Autodesk Fusion 360 part; units mm, degrees
(part 4 of 12)
  spline S130 degree 5 poles (-15.9343, -68.6757) (-15.9205, -68.6585) (-15.8929, -68.6243) (-15.8515, -68.5729) (-15.7966, -68.5042) (-15.7284, -68.4182) (-15.6605, -68.332) (-15.593, -68.2456) (-15.5259, -68.1591) (-15.4592, -68.0723) (-15.3928, -67.9855) (-15.3269, -67.8984) (-15.2613, -67.8111) (-15.1961, -67.7237) (-15.1313, -67.6361) (-15.0669, -67.5484) (-15.0029, -67.4604) (-14.9393, -67.3723) (-14.8761, -67.284) (-14.8134, -67.1956) (-14.751, -67.1069) (-14.6891, -67.0181) (-14.6276, -66.9291) (-14.5665, -66.8399) (-14.5059, -66.7506) (-14.4456, -66.6611) (-14.3859, -66.5714) (-14.3265, -66.4815) (-14.2676, -66.3914) (-14.2092, -66.3012) (-14.1512, -66.2108) (-14.0937, -66.1202) (-14.0367, -66.0294) (-13.9801, -65.9385) (-13.924, -65.8473) (-13.8684, -65.756) (-13.8133, -65.6645) (-13.7587, -65.5728) (-13.7046, -65.481) (-13.651, -65.3889) (-13.5979, -65.2967) (-13.5453, -65.2043) (-13.4933, -65.1117) (-13.4418, -65.0189) (-13.3909, -64.9259) (-13.3405, -64.8327) (-13.2907, -64.7393) (-13.2415, -64.6458) (-13.1928, -64.552) (-13.1448, -64.4581) (-13.0974, -64.3639) (-13.0506, -64.2695) (-13.0044, -64.175) (-12.9589, -64.0802) (-12.9141, -63.9852) (-12.873, -63.8968) (-12.8413, -63.8272) (-12.8185, -63.7766) (-12.8044, -63.745) (-12.7989, -63.7326) knots -1 -1 -1 -1 -1 -1 -0.985714 -0.971429 -0.957143 -0.942857 -0.928571 -0.914286 -0.9 -0.885714 -0.871429 -0.857143 -0.842857 -0.828571 -0.814286 -0.8 -0.785714 -0.771429 -0.757143 -0.742857 -0.728571 -0.714286 -0.7 -0.685714 -0.671429 -0.657143 -0.642857 -0.628571 -0.614286 -0.6 -0.585714 -0.571429 -0.557143 -0.542857 -0.528571 -0.514286 -0.5 -0.485714 -0.471429 -0.457143 -0.442857 -0.428571 -0.414286 -0.4 -0.385714 -0.371429 -0.357143 -0.342857 -0.328571 -0.314286 -0.3 -0.285714 -0.271429 -0.257143 -0.242857 -0.228571 -0.21931 -0.21931 -0.21931 -0.21931 -0.21931 -0.21931
  spline S131 degree 3 poles (-11.166, -62.8653) (-11.3583, -62.8311) (-11.5555, -62.8348) (-11.9372, -62.9176) (-12.1182, -62.9959) (-12.3924, -63.1847) (-12.4944, -63.278) (-12.6701, -63.4896) (-12.743, -63.607) (-12.7989, -63.7326) knots 0 0 0 0 0.058597 0.058597 0.117193 0.117193 0.158456 0.158456 0.199718 0.199718 0.199718 0.199718
  arc A66 (-11.166, -62.8653) -> (-11.0086, -62.893) centre (0, 0) ccw
  spline S132 degree 3 poles (-9.7708, -64.2666) (-9.7843, -64.0717) (-9.8358, -63.8814) (-10.0088, -63.5311) (-10.1287, -63.3746) (-10.3784, -63.1545) (-10.4935, -63.0781) (-10.7415, -62.959) (-10.8731, -62.9167) (-11.0086, -62.893) knots 0 0 0 0 0.058597 0.058597 0.117193 0.117193 0.158456 0.158456 0.199718 0.199718 0.199718 0.199718
  spline S133 degree 5 poles (-9.7708, -64.2666) (-9.7698, -64.2801) (-9.7674, -64.3146) (-9.7633, -64.3699) (-9.7573, -64.4461) (-9.749, -64.5433) (-9.7393, -64.6479) (-9.729, -64.7525) (-9.7179, -64.8572) (-9.7062, -64.9618) (-9.6939, -65.0665) (-9.6809, -65.1713) (-9.6673, -65.276) (-9.653, -65.3808) (-9.6381, -65.4855) (-9.6227, -65.5903) (-9.6066, -65.6951) (-9.5899, -65.7999) (-9.5727, -65.9048) (-9.555, -66.0096) (-9.5366, -66.1144) (-9.5177, -66.2192) (-9.4983, -66.3241) (-9.4783, -66.4289) (-9.4578, -66.5337) (-9.4368, -66.6386) (-9.4153, -66.7434) (-9.3932, -66.8482) (-9.3707, -66.953) (-9.3476, -67.0578) (-9.3241, -67.1626) (-9.3, -67.2674) (-9.2755, -67.3721) (-9.2505, -67.4769) (-9.225, -67.5816) (-9.199, -67.6863) (-9.1726, -67.791) (-9.1457, -67.8957) (-9.1183, -68.0004) (-9.0905, -68.105) (-9.0622, -68.2097) (-9.0335, -68.3143) (-9.0043, -68.4188) (-8.9747, -68.5234) (-8.9447, -68.6279) (-8.9142, -68.7324) (-8.8832, -68.8369) (-8.8519, -68.9413) (-8.8201, -69.0457) (-8.7879, -69.1501) (-8.7552, -69.2544) (-8.7222, -69.3587) (-8.6887, -69.463) (-8.6548, -69.5673) (-8.6205, -69.6715) (-8.5858, -69.7756) (-8.5577, -69.859) (-8.5365, -69.9214) (-8.5222, -69.9631) (-8.5151, -69.9839) knots 0.21931 0.21931 0.21931 0.21931 0.21931 0.21931 0.228571 0.242857 0.257143 0.271429 0.285714 0.3 0.314286 0.328571 0.342857 0.357143 0.371429 0.385714 0.4 0.414286 0.428571 0.442857 0.457143 0.471429 0.485714 0.5 0.514286 0.528571 0.542857 0.557143 0.571429 0.585714 0.6 0.614286 0.628571 0.642857 0.657143 0.671429 0.685714 0.7 0.714286 0.728571 0.742857 0.757143 0.771429 0.785714 0.8 0.814286 0.828571 0.842857 0.857143 0.871429 0.885714 0.9 0.914286 0.928571 0.942857 0.957143 0.971429 0.985714 1 1 1 1 1 1
  arc A67 (-8.5151, -69.9839) -> (-6.2215, -70.2249) centre (0, 0) ccw
  spline S134 degree 5 poles (-6.2215, -70.2249) (-6.2101, -70.2061) (-6.1875, -70.1683) (-6.1538, -70.1116) (-6.109, -70.036) (-6.0534, -69.9413) (-5.9981, -69.8465) (-5.9433, -69.7516) (-5.8889, -69.6565) (-5.8349, -69.5614) (-5.7813, -69.4661) (-5.7281, -69.3707) (-5.6753, -69.2752) (-5.6229, -69.1795) (-5.5709, -69.0838) (-5.5194, -68.9879) (-5.4682, -68.8919) (-5.4175, -68.7958) (-5.3672, -68.6996) (-5.3174, -68.6032) (-5.268, -68.5068) (-5.219, -68.4102) (-5.1705, -68.3135) (-5.1224, -68.2167) (-5.0748, -68.1198) (-5.0276, -68.0228) (-4.9809, -67.9256) (-4.9347, -67.8284) (-4.8889, -67.731) (-4.8436, -67.6335) (-4.7988, -67.5359) (-4.7544, -67.4382) (-4.7106, -67.3404) (-4.6672, -67.2424) (-4.6243, -67.1444) (-4.582, -67.0462) (-4.5401, -66.9479) (-4.4988, -66.8495) (-4.458, -66.751) (-4.4177, -66.6524) (-4.378, -66.5537) (-4.3388, -66.4549) (-4.3002, -66.3559) (-4.2621, -66.2569) (-4.2246, -66.1577) (-4.1877, -66.0584) (-4.1514, -65.959) (-4.1156, -65.8595) (-4.0805, -65.7599) (-4.0461, -65.6602) (-4.0122, -65.5603) (-3.979, -65.4604) (-3.9464, -65.3603) (-3.9145, -65.2601) (-3.8833, -65.1598) (-3.855, -65.0665) (-3.8333, -64.9932) (-3.8178, -64.9399) (-3.8082, -64.9067) (-3.8045, -64.8937) knots -1 -1 -1 -1 -1 -1 -0.985714 -0.971429 -0.957143 -0.942857 -0.928571 -0.914286 -0.9 -0.885714 -0.871429 -0.857143 -0.842857 -0.828571 -0.814286 -0.8 -0.785714 -0.771429 -0.757143 -0.742857 -0.728571 -0.714286 -0.7 -0.685714 -0.671429 -0.657143 -0.642857 -0.628571 -0.614286 -0.6 -0.585714 -0.571429 -0.557143 -0.542857 -0.528571 -0.514286 -0.5 -0.485714 -0.471429 -0.457143 -0.442857 -0.428571 -0.414286 -0.4 -0.385714 -0.371429 -0.357143 -0.342857 -0.328571 -0.314286 -0.3 -0.285714 -0.271429 -0.257143 -0.242857 -0.228571 -0.21931 -0.21931 -0.21931 -0.21931 -0.21931 -0.21931
  spline S135 degree 3 poles (-2.3082, -63.8075) (-2.5034, -63.8004) (-2.6981, -63.8315) (-3.0646, -63.9667) (-3.2329, -64.0694) (-3.4781, -64.2945) (-3.5662, -64.401) (-3.7108, -64.635) (-3.7667, -64.7614) (-3.8045, -64.8937) knots 0 0 0 0 0.058597 0.058597 0.117193 0.117193 0.158456 0.158456 0.199718 0.199718 0.199718 0.199718
  arc A68 (-2.3082, -63.8075) -> (-2.1484, -63.813) centre (0, 0) ccw
  spline S136 degree 3 poles (-0.7315, -65.001) (-0.772, -64.8099) (-0.8495, -64.6286) (-1.0696, -64.3058) (-1.2101, -64.1675) (-1.488, -63.9842) (-1.6126, -63.9247) (-1.8748, -63.8412) (-2.0109, -63.8177) (-2.1484, -63.813) knots 0 0 0 0 0.058597 0.058597 0.117193 0.117193 0.158456 0.158456 0.199718 0.199718 0.199718 0.199718
  spline S137 degree 5 poles (-0.7315, -65.001) (-0.7287, -65.0143) (-0.7215, -65.048) (-0.7097, -65.1022) (-0.6932, -65.1769) (-0.6714, -65.272) (-0.6473, -65.3742) (-0.6225, -65.4764) (-0.597, -65.5785) (-0.5708, -65.6805) (-0.544, -65.7824) (-0.5166, -65.8843) (-0.4885, -65.9862) (-0.4598, -66.0879) (-0.4305, -66.1896) (-0.4006, -66.2912) (-0.3701, -66.3928) (-0.339, -66.4942) (-0.3074, -66.5956) (-0.2752, -66.697) (-0.2425, -66.7982) (-0.2092, -66.8994) (-0.1753, -67.0005) (-0.141, -67.1016) (-0.1061, -67.2025) (-0.0707, -67.3034) (-0.0348, -67.4042) (0.0017, -67.5049) (0.0386, -67.6056) (0.076, -67.7061) (0.1139, -67.8066) (0.1523, -67.907) (0.1912, -68.0074) (0.2305, -68.1076) (0.2703, -68.2078) (0.3106, -68.3079) (0.3514, -68.4079) (0.3926, -68.5078) (0.4343, -68.6076) (0.4764, -68.7074) (0.5189, -68.8071) (0.5619, -68.9066) (0.6054, -69.0061) (0.6492, -69.1055) (0.6936, -69.2049) (0.7383, -69.3041) (0.7835, -69.4032) (0.829, -69.5023) (0.8751, -69.6013) (0.9215, -69.7002) (0.9683, -69.7989) (1.0156, -69.8976) (1.0632, -69.9962) (1.1113, -70.0948) (1.1598, -70.1932) (1.2086, -70.2915) (1.248, -70.3701) (1.2778, -70.429) (1.2977, -70.4683) (1.3077, -70.4879) knots 0.21931 0.21931 0.21931 0.21931 0.21931 0.21931 0.228571 0.242857 0.257143 0.271429 0.285714 0.3 0.314286 0.328571 0.342857 0.357143 0.371429 0.385714 0.4 0.414286 0.428571 0.442857 0.457143 0.471429 0.485714 0.5 0.514286 0.528571 0.542857 0.557143 0.571429 0.585714 0.6 0.614286 0.628571 0.642857 0.657143 0.671429 0.685714 0.7 0.714286 0.728571 0.742857 0.757143 0.771429 0.785714 0.8 0.814286 0.828571 0.842857 0.857143 0.871429 0.885714 0.9 0.914286 0.928571 0.942857 0.957143 0.971429 0.985714 1 1 1 1 1 1
  arc A69 (1.3077, -70.4879) -> (3.6125, -70.4074) centre (0, 0) ccw
  spline S138 degree 5 poles (3.6125, -70.4074) (3.6211, -70.3871) (3.6382, -70.3466) (3.6638, -70.2857) (3.6976, -70.2046) (3.7395, -70.1031) (3.781, -70.0015) (3.8221, -69.8999) (3.8627, -69.7982) (3.903, -69.6965) (3.9428, -69.5946) (3.9822, -69.4928) (4.0212, -69.3908) (4.0598, -69.2888) (4.0979, -69.1868) (4.1356, -69.0847) (4.1729, -68.9825) (4.2097, -68.8803) (4.2461, -68.778) (4.2821, -68.6756) (4.3176, -68.5733) (4.3526, -68.4708) (4.3872, -68.3683) (4.4214, -68.2658) (4.455, -68.1632) (4.4882, -68.0605) (4.521, -67.9578) (4.5532, -67.855) (4.585, -67.7522) (4.6163, -67.6494) (4.6471, -67.5465) (4.6774, -67.4436) (4.7072, -67.3406) (4.7366, -67.2376) (4.7654, -67.1345) (4.7936, -67.0314) (4.8214, -66.9283) (4.8486, -66.8251) (4.8753, -66.7219) (4.9015, -66.6186) (4.9271, -66.5153) (4.9521, -66.412) (4.9766, -66.3086) (5.0005, -66.2052) (5.0239, -66.1018) (5.0466, -65.9983) (5.0688, -65.8949) (5.0903, -65.7913) (5.1112, -65.6878) (5.1314, -65.5843) (5.1511, -65.4807) (5.17, -65.3771) (5.1884, -65.2735) (5.206, -65.1698) (5.2229, -65.0662) (5.238, -64.9698) (5.2493, -64.8941) (5.2573, -64.8392) (5.2621, -64.805) (5.264, -64.7916) knots -1 -1 -1 -1 -1 -1 -0.985714 -0.971429 -0.957143 -0.942857 -0.928571 -0.914286 -0.9 -0.885714 -0.871429 -0.857143 -0.842857 -0.828571 -0.814286 -0.8 -0.785714 -0.771429 -0.757143 -0.742857 -0.728571 -0.714286 -0.7 -0.685714 -0.671429 -0.657143 -0.642857 -0.628571 -0.614286 -0.6 -0.585714 -0.571429 -0.557143 -0.542857 -0.528571 -0.514286 -0.5 -0.485714 -0.471429 -0.457143 -0.442857 -0.428571 -0.414286 -0.4 -0.385714 -0.371429 -0.357143 -0.342857 -0.328571 -0.314286 -0.3 -0.285714 -0.271429 -0.257143 -0.242857 -0.228571 -0.21931 -0.21931 -0.21931 -0.21931 -0.21931 -0.21931
  spline S139 degree 3 poles (6.5945, -63.5077) (6.4003, -63.5279) (6.2118, -63.5858) (5.8676, -63.7707) (5.7153, -63.8958) (5.5038, -64.1529) (5.4314, -64.2706) (5.3208, -64.5225) (5.2831, -64.6554) (5.264, -64.7916) knots 0 0 0 0 0.058597 0.058597 0.117193 0.117193 0.158456 0.158456 0.199718 0.199718 0.199718 0.199718
  arc A70 (6.5945, -63.5077) -> (6.7536, -63.491) centre (0, 0) ccw
  spline S140 degree 3 poles (8.322, -64.4702) (8.2553, -64.2866) (8.1533, -64.1178) (7.8905, -63.8288) (7.7321, -63.7114) (7.4314, -63.5686) (7.2996, -63.527) (7.0285, -63.4808) (6.8903, -63.4765) (6.7536, -63.491) knots 0 0 0 0 0.058597 0.058597 0.117193 0.117193 0.158456 0.158456 0.199718 0.199718 0.199718 0.199718
  spline S141 degree 5 poles (8.322, -64.4702) (8.3266, -64.483) (8.3385, -64.5154) (8.3576, -64.5674) (8.3844, -64.6391) (8.4192, -64.7302) (8.4573, -64.8281) (8.4961, -64.9258) (8.5356, -65.0233) (8.5757, -65.1207) (8.6164, -65.218) (8.6578, -65.3151) (8.6997, -65.412) (8.7423, -65.5087) (8.7855, -65.6054) (8.8292, -65.7018) (8.8736, -65.7981) (8.9185, -65.8943) (8.9639, -65.9903) (9.0099, -66.0862) (9.0564, -66.1819) (9.1035, -66.2775) (9.151, -66.3729) (9.1991, -66.4681) (9.2477, -66.5633) (9.2968, -66.6582) (9.3464, -66.7531) (9.3965, -66.8477) (9.4471, -66.9423) (9.4981, -67.0367) (9.5497, -67.1309) (9.6017, -67.225) (9.6541, -67.3189) (9.707, -67.4127) (9.7604, -67.5064) (9.8142, -67.5999) (9.8685, -67.6932) (9.9232, -67.7864) (9.9784, -67.8795) (10.034, -67.9724) (10.09, -68.0652) (10.1464, -68.1578) (10.2033, -68.2503) (10.2606, -68.3427) (10.3183, -68.4348) (10.3764, -68.5269) (10.4349, -68.6188) (10.4938, -68.7105) (10.5532, -68.8021) (10.6129, -68.8936) (10.673, -68.9849) (10.7336, -69.0761) (10.7945, -69.1671) (10.8558, -69.2579) (10.9175, -69.3487) (10.9795, -69.4392) (11.0295, -69.5116) (11.0672, -69.5658) (11.0923, -69.6019) (11.105, -69.6199) knots 0.21931 0.21931 0.21931 0.21931 0.21931 0.21931 0.228571 0.242857 0.257143 0.271429 0.285714 0.3 0.314286 0.328571 0.342857 0.357143 0.371429 0.385714 0.4 0.414286 0.428571 0.442857 0.457143 0.471429 0.485714 0.5 0.514286 0.528571 0.542857 0.557143 0.571429 0.585714 0.6 0.614286 0.628571 0.642857 0.657143 0.671429 0.685714 0.7 0.714286 0.728571 0.742857 0.757143 0.771429 0.785714 0.8 0.814286 0.828571 0.842857 0.857143 0.871429 0.885714 0.9 0.914286 0.928571 0.942857 0.957143 0.971429 0.985714 1 1 1 1 1 1
  arc A71 (11.105, -69.6199) -> (13.3762, -69.2194) centre (0, 0) ccw
  spline S142 degree 5 poles (13.3762, -69.2194) (13.3818, -69.1982) (13.3932, -69.1556) (13.41, -69.0918) (13.4322, -69.0068) (13.4596, -68.9004) (13.4865, -68.7941) (13.513, -68.6877) (13.5392, -68.5814) (13.5649, -68.475) (13.5901, -68.3686) (13.615, -68.2623) (13.6394, -68.1559) (13.6634, -68.0495) (13.687, -67.9431) (13.7101, -67.8368) (13.7328, -67.7304) (13.755, -67.624) (13.7768, -67.5177) (13.7982, -67.4113) (13.8191, -67.305) (13.8396, -67.1987) (13.8596, -67.0924) (13.8791, -66.9861) (13.8982, -66.8798) (13.9168, -66.7735) (13.9349, -66.6672) (13.9525, -66.561) (13.9697, -66.4548) (13.9864, -66.3486) (14.0026, -66.2424) (14.0182, -66.1362) (14.0334, -66.0301) (14.0481, -65.924) (14.0623, -65.818) (14.076, -65.7119) (14.0891, -65.6059) (14.1017, -65.4999) (14.1138, -65.394) (14.1253, -65.2881) (14.1363, -65.1823) (14.1467, -65.0765) (14.1566, -64.9707) (14.1659, -64.865) (14.1746, -64.7593) (14.1827, -64.6537) (14.1902, -64.5481) (14.1971, -64.4426) (14.2034, -64.3372) (14.2091, -64.2318) (14.2141, -64.1265) (14.2185, -64.0213) (14.2222, -63.9161) (14.2252, -63.8111) (14.2276, -63.706) (14.2291, -63.6085) (14.2298, -63.532) (14.23, -63.4765) (14.23, -63.442) (14.23, -63.4285) knots -1 -1 -1 -1 -1 -1 -0.985714 -0.971429 -0.957143 -0.942857 -0.928571 -0.914286 -0.9 -0.885714 -0.871429 -0.857143 -0.842857 -0.828571 -0.814286 -0.8 -0.785714 -0.771429 -0.757143 -0.742857 -0.728571 -0.714286 -0.7 -0.685714 -0.671429 -0.657143 -0.642857 -0.628571 -0.614286 -0.6 -0.585714 -0.571429 -0.557143 -0.542857 -0.528571 -0.514286 -0.5 -0.485714 -0.471429 -0.457143 -0.442857 -0.428571 -0.414286 -0.4 -0.385714 -0.371429 -0.357143 -0.342857 -0.328571 -0.314286 -0.3 -0.285714 -0.271429 -0.257143 -0.242857 -0.228571 -0.21931 -0.21931 -0.21931 -0.21931 -0.21931 -0.21931
  spline S143 degree 3 poles (15.3689, -61.9719) (15.1794, -62.0189) (15.0008, -62.1025) (14.6857, -62.3334) (14.5522, -62.4786) (14.3786, -62.7626) (14.3233, -62.8892) (14.2488, -63.154) (14.2299, -63.2909) (14.23, -63.4285) knots 0 0 0 0 0.058597 0.058597 0.117193 0.117193 0.158456 0.158456 0.199718 0.199718 0.199718 0.199718
  arc A72 (15.3689, -61.9719) -> (15.5241, -61.9332) centre (0, 0) ccw
  spline S144 degree 3 poles (17.2135, -62.6846) (17.1219, -62.5121) (16.9975, -62.3591) (16.697, -62.1095) (16.5238, -62.0153) (16.2061, -61.9157) (16.0698, -61.8928) (15.7949, -61.8848) (15.6575, -61.8998) (15.5241, -61.9332) knots 0 0 0 0 0.058597 0.058597 0.117193 0.117193 0.158456 0.158456 0.199718 0.199718 0.199718 0.199718
  spline S145 degree 5 poles (17.2135, -62.6846) (17.2199, -62.6966) (17.2361, -62.727) (17.2624, -62.7759) (17.2989, -62.8431) (17.346, -62.9285) (17.3973, -63.0202) (17.4494, -63.1115) (17.502, -63.2026) (17.5553, -63.2935) (17.6092, -63.3841) (17.6636, -63.4745) (17.7187, -63.5646) (17.7743, -63.6545) (17.8305, -63.7442) (17.8872, -63.8336) (17.9446, -63.9228) (18.0024, -64.0118) (18.0608, -64.1006) (18.1196, -64.1891) (18.179, -64.2774) (18.2389, -64.3655) (18.2993, -64.4534) (18.3602, -64.541) (18.4215, -64.6284) (18.4834, -64.7157) (18.5457, -64.8027) (18.6085, -64.8894) (18.6717, -64.976) (18.7354, -65.0624) (18.7995, -65.1485) (18.8641, -65.2345) (18.9291, -65.3202) (18.9946, -65.4057) (19.0605, -65.491) (19.1268, -65.5761) (19.1935, -65.661) (19.2607, -65.7457) (19.3283, -65.8302) (19.3962, -65.9145) (19.4646, -65.9986) (19.5334, -66.0824) (19.6026, -66.1661) (19.6722, -66.2496) (19.7421, -66.3328) (19.8125, -66.4159) (19.8832, -66.4987) (19.9544, -66.5814) (20.0259, -66.6638) (20.0978, -66.7461) (20.17, -66.8281) (20.2426, -66.91) (20.3156, -66.9916) (20.389, -67.0731) (20.4627, -67.1543) (20.5368, -67.2354) (20.5963, -67.3001) (20.6411, -67.3485) (20.6711, -67.3807) (20.6861, -67.3969) knots 0.21931 0.21931 0.21931 0.21931 0.21931 0.21931 0.228571 0.242857 0.257143 0.271429 0.285714 0.3 0.314286 0.328571 0.342857 0.357143 0.371429 0.385714 0.4 0.414286 0.428571 0.442857 0.457143 0.471429 0.485714 0.5 0.514286 0.528571 0.542857 0.557143 0.571429 0.585714 0.6 0.614286 0.628571 0.642857 0.657143 0.671429 0.685714 0.7 0.714286 0.728571 0.742857 0.757143 0.771429 0.785714 0.8 0.814286 0.828571 0.842857 0.857143 0.871429 0.885714 0.9 0.914286 0.928571 0.942857 0.957143 0.971429 0.985714 1 1 1 1 1 1
  arc A73 (20.6861, -67.3969) -> (22.8795, -66.6842) centre (0, 0) ccw
  spline S146 degree 5 poles (22.8795, -66.6842) (22.8821, -66.6623) (22.8874, -66.6186) (22.8952, -66.5531) (22.9054, -66.4658) (22.9177, -66.3567) (22.9295, -66.2476) (22.941, -66.1386) (22.9521, -66.0296) (22.9627, -65.9207) (22.9729, -65.8119) (22.9828, -65.7031) (22.9921, -65.5944) (23.0011, -65.4857) (23.0096, -65.3771) (23.0177, -65.2685) (23.0254, -65.16) (23.0326, -65.0516) (23.0394, -64.9433) (23.0458, -64.835) (23.0517, -64.7268) (23.0571, -64.6186) (23.0621, -64.5106) (23.0667, -64.4026) (23.0708, -64.2947) (23.0744, -64.1868) (23.0776, -64.0791) (23.0802, -63.9714) (23.0825, -63.8638) (23.0842, -63.7564) (23.0854, -63.649) (23.0862, -63.5417) (23.0865, -63.4344) (23.0863, -63.3273) (23.0855, -63.2203) (23.0843, -63.1134) (23.0826, -63.0066) (23.0803, -62.8999) (23.0775, -62.7933) (23.0742, -62.6869) (23.0703, -62.5805) (23.0659, -62.4743) (23.061, -62.3682) (23.0555, -62.2622) (23.0494, -62.1564) (23.0427, -62.0506) (23.0355, -61.9451) (23.0276, -61.8396) (23.0192, -61.7343) (23.0101, -61.6292) (23.0004, -61.5242) (22.9901, -61.4194) (22.9792, -61.3148) (22.9676, -61.2103) (22.9553, -61.106) (22.9432, -61.0092) (22.9332, -60.9333) (22.9257, -60.8784) (22.9209, -60.8442) (22.919, -60.8307) knots -1 -1 -1 -1 -1 -1 -0.985714 -0.971429 -0.957143 -0.942857 -0.928571 -0.914286 -0.9 -0.885714 -0.871429 -0.857143 -0.842857 -0.828571 -0.814286 -0.8 -0.785714 -0.771429 -0.757143 -0.742857 -0.728571 -0.714286 -0.7 -0.685714 -0.671429 -0.657143 -0.642857 -0.628571 -0.614286 -0.6 -0.585714 -0.571429 -0.557143 -0.542857 -0.528571 -0.514286 -0.5 -0.485714 -0.471429 -0.457143 -0.442857 -0.428571 -0.414286 -0.4 -0.385714 -0.371429 -0.357143 -0.342857 -0.328571 -0.314286 -0.3 -0.285714 -0.271429 -0.257143 -0.242857 -0.228571 -0.21931 -0.21931 -0.21931 -0.21931 -0.21931 -0.21931
  spline S147 degree 3 poles (23.8442, -59.2299) (23.663, -59.3028) (23.4978, -59.4104) (23.2179, -59.683) (23.1059, -59.8453) (22.9735, -60.1506) (22.9364, -60.2838) (22.8995, -60.5564) (22.8998, -60.6945) (22.919, -60.8307) knots 0 0 0 0 0.058597 0.058597 0.117193 0.117193 0.158456 0.158456 0.199718 0.199718 0.199718 0.199718
  arc A74 (23.8442, -59.2299) -> (23.9924, -59.17) centre (0, 0) ccw
  spline S148 degree 3 poles (25.77, -59.6789) (25.6553, -59.5208) (25.5108, -59.3867) (25.1784, -59.1813) (24.9938, -59.1121) (24.6654, -59.0577) (24.5273, -59.054) (24.2539, -59.0844) (24.1199, -59.1183) (23.9924, -59.17) knots 0 0 0 0 0.058597 0.058597 0.117193 0.117193 0.158456 0.158456 0.199718 0.199718 0.199718 0.199718
  spline S149 degree 5 poles (25.77, -59.6789) (25.778, -59.6899) (25.7983, -59.7178) (25.8311, -59.7625) (25.8766, -59.824) (25.9351, -59.902) (25.9987, -59.9856) (26.063, -60.0688) (26.1278, -60.1517) (26.1932, -60.2343) (26.2591, -60.3165) (26.3257, -60.3984) (26.3927, -60.4801) (26.4603, -60.5613) (26.5284, -60.6423) (26.5971, -60.723) (26.6663, -60.8033) (26.7359, -60.8834) (26.8061, -60.9632) (26.8767, -61.0427) (26.9478, -61.1218) (27.0194, -61.2007) (27.0914, -61.2793) (27.1639, -61.3577) (27.2368, -61.4357) (27.3102, -61.5135) (27.384, -61.5909) (27.4582, -61.6681) (27.5329, -61.7451) (27.608, -61.8217) (27.6835, -61.8981) (27.7594, -61.9742) (27.8357, -62.0501) (27.9125, -62.1256) (27.9896, -62.201) (28.0671, -62.276) (28.145, -62.3508) (28.2233, -62.4253) (28.302, -62.4996) (28.381, -62.5736) (28.4604, -62.6473) (28.5402, -62.7208) (28.6204, -62.794) (28.7009, -62.867) (28.7817, -62.9397) (28.863, -63.0122) (28.9446, -63.0844) (29.0265, -63.1563) (29.1088, -63.228) (29.1914, -63.2995) (29.2744, -63.3707) (29.3577, -63.4416) (29.4413, -63.5123) (29.5253, -63.5827) (29.6096, -63.6529) (29.6943, -63.7229) (29.7622, -63.7787) (29.8134, -63.8204) (29.8475, -63.8481) (29.8646, -63.862) knots 0.21931 0.21931 0.21931 0.21931 0.21931 0.21931 0.228571 0.242857 0.257143 0.271429 0.285714 0.3 0.314286 0.328571 0.342857 0.357143 0.371429 0.385714 0.4 0.414286 0.428571 0.442857 0.457143 0.471429 0.485714 0.5 0.514286 0.528571 0.542857 0.557143 0.571429 0.585714 0.6 0.614286 0.628571 0.642857 0.657143 0.671429 0.685714 0.7 0.714286 0.728571 0.742857 0.757143 0.771429 0.785714 0.8 0.814286 0.828571 0.842857 0.857143 0.871429 0.885714 0.9 0.914286 0.928571 0.942857 0.957143 0.971429 0.985714 1 1 1 1 1 1
  arc A75 (29.8646, -63.862) -> (31.9375, -62.851) centre (0, 0) ccw
  spline S150 degree 5 poles (31.9375, -62.851) (31.9371, -62.829) (31.9362, -62.785) (31.9348, -62.719) (31.9327, -62.6311) (31.9297, -62.5214) (31.9263, -62.4117) (31.9225, -62.3022) (31.9183, -62.1927) (31.9136, -62.0834) (31.9086, -61.9742) (31.9032, -61.8651) (31.8974, -61.7561) (31.8911, -61.6472) (31.8844, -61.5385) (31.8773, -61.4299) (31.8698, -61.3214) (31.8619, -61.213) (31.8536, -61.1048) (31.8448, -60.9966) (31.8356, -60.8887) (31.8259, -60.7808) (31.8158, -60.6731) (31.8053, -60.5655) (31.7943, -60.4581) (31.7829, -60.3508) (31.771, -60.2437) (31.7587, -60.1367) (31.7459, -60.0299) (31.7327, -59.9232) (31.719, -59.8167) (31.7048, -59.7103) (31.6902, -59.6041) (31.675, -59.498) (31.6594, -59.3922) (31.6433, -59.2865) (31.6267, -59.181) (31.6097, -59.0756) (31.5921, -58.9705) (31.5739, -58.8655) (31.5553, -58.7607) (31.5362, -58.6561) (31.5165, -58.5518) (31.4963, -58.4476) (31.4756, -58.3436) (31.4543, -58.2398) (31.4324, -58.1363) (31.41, -58.033) (31.3869, -57.9299) (31.3633, -57.8271) (31.3391, -57.7244) (31.3143, -57.6221) (31.2889, -57.52) (31.2629, -57.4181) (31.2362, -57.3165) (31.2108, -57.2224) (31.1903, -57.1487) (31.1752, -57.0953) (31.1657, -57.0621) (31.162, -57.049) knots -1 -1 -1 -1 -1 -1 -0.985714 -0.971429 -0.957143 -0.942857 -0.928571 -0.914286 -0.9 -0.885714 -0.871429 -0.857143 -0.842857 -0.828571 -0.814286 -0.8 -0.785714 -0.771429 -0.757143 -0.742857 -0.728571 -0.714286 -0.7 -0.685714 -0.671429 -0.657143 -0.642857 -0.628571 -0.614286 -0.6 -0.585714 -0.571429 -0.557143 -0.542857 -0.528571 -0.514286 -0.5 -0.485714 -0.471429 -0.457143 -0.442857 -0.428571 -0.414286 -0.4 -0.385714 -0.371429 -0.357143 -0.342857 -0.328571 -0.314286 -0.3 -0.285714 -0.271429 -0.257143 -0.242857 -0.228571 -0.21931 -0.21931 -0.21931 -0.21931 -0.21931 -0.21931
  spline S151 degree 3 poles (31.8553, -55.335) (31.6861, -55.4324) (31.5374, -55.562) (31.2982, -55.8708) (31.2099, -56.0471) (31.1213, -56.368) (31.103, -56.505) (31.1044, -56.78) (31.124, -56.9168) (31.162, -57.049) knots 0 0 0 0 0.058597 0.058597 0.117193 0.117193 0.158456 0.158456 0.199718 0.199718 0.199718 0.199718
  arc A76 (31.8553, -55.335) -> (31.9938, -55.255) centre (0, 0) ccw
  spline S152 degree 3 poles (33.8249, -55.5116) (33.6893, -55.371) (33.5275, -55.2583) (33.1698, -55.1012) (32.9774, -55.0583) (32.6446, -55.0502) (32.5073, -55.0658) (32.2408, -55.1339) (32.1128, -55.1861) (31.9938, -55.255) knots 0 0 0 0 0.058597 0.058597 0.117193 0.117193 0.158456 0.158456 0.199718 0.199718 0.199718 0.199718
  spline S153 degree 5 poles (33.8249, -55.5116) (33.8343, -55.5214) (33.8583, -55.5462) (33.897, -55.5859) (33.9506, -55.6405) (34.0195, -55.7096) (34.0941, -55.7835) (34.1693, -55.857) (34.245, -55.93) (34.3213, -56.0027) (34.398, -56.075) (34.4753, -56.1468) (34.5531, -56.2183) (34.6313, -56.2894) (34.7101, -56.3601) (34.7893, -56.4304) (34.8689, -56.5004) (34.9491, -56.57) (35.0296, -56.6392) (35.1106, -56.7081) (35.1921, -56.7766) (35.2739, -56.8448) (35.3562, -56.9126) (35.4389, -56.98) (35.5219, -57.0472) (35.6054, -57.114) (35.6893, -57.1804) (35.7736, -57.2465) (35.8582, -57.3123) (35.9432, -57.3778) (36.0286, -57.4429) (36.1144, -57.5077) (36.2005, -57.5722) (36.287, -57.6364) (36.3739, -57.7002) (36.4611, -57.7638) (36.5486, -57.827) (36.6365, -57.8899) (36.7248, -57.9525) (36.8134, -58.0147) (36.9023, -58.0767) (36.9915, -58.1384) (37.0811, -58.1997) (37.1709, -58.2608) (37.2612, -58.3215) (37.3517, -58.382) (37.4425, -58.4421) (37.5337, -58.502) (37.6251, -58.5615) (37.7169, -58.6208) (37.809, -58.6797) (37.9014, -58.7384) (37.994, -58.7968) (38.087, -58.8548) (38.1802, -58.9126) (38.2738, -58.9701) (38.3489, -59.0159) (38.4053, -59.0501) (38.443, -59.0728) (38.4618, -59.0842) knots 0.21931 0.21931 0.21931 0.21931 0.21931 0.21931 0.228571 0.242857 0.257143 0.271429 0.285714 0.3 0.314286 0.328571 0.342857 0.357143 0.371429 0.385714 0.4 0.414286 0.428571 0.442857 0.457143 0.471429 0.485714 0.5 0.514286 0.528571 0.542857 0.557143 0.571429 0.585714 0.6 0.614286 0.628571 0.642857 0.657143 0.671429 0.685714 0.7 0.714286 0.728571 0.742857 0.757143 0.771429 0.785714 0.8 0.814286 0.828571 0.842857 0.857143 0.871429 0.885714 0.9 0.914286 0.928571 0.942857 0.957143 0.971429 0.985714 1 1 1 1 1 1
  arc A77 (38.4618, -59.0842) -> (40.3738, -57.7945) centre (0, 0) ccw
  spline S154 degree 5 poles (40.3738, -57.7945) (40.3703, -57.7728) (40.3634, -57.7293) (40.3528, -57.6642) (40.3385, -57.5774) (40.3203, -57.4692) (40.3016, -57.3611) (40.2826, -57.2531) (40.2632, -57.1453) (40.2434, -57.0377) (40.2232, -56.9302) (40.2027, -56.823) (40.1817, -56.7158) (40.1604, -56.6089) (40.1386, -56.5022) (40.1165, -56.3956) (40.094, -56.2892) (40.071, -56.183) (40.0477, -56.0769) (40.024, -55.9711) (39.9998, -55.8654) (39.9752, -55.76) (39.9503, -55.6547) (39.9249, -55.5497) (39.8991, -55.4448) (39.8728, -55.3402) (39.8462, -55.2357) (39.8191, -55.1315) (39.7915, -55.0275) (39.7636, -54.9237) (39.7352, -54.8201) (39.7063, -54.7167) (39.6771, -54.6136) (39.6473, -54.5107) (39.6171, -54.408) (39.5865, -54.3056) (39.5554, -54.2034) (39.5238, -54.1015) (39.4917, -53.9998) (39.4592, -53.8984) (39.4261, -53.7972) (39.3926, -53.6963) (39.3586, -53.5957) (39.3241, -53.4953) (39.2891, -53.3953) (39.2536, -53.2955) (39.2175, -53.196) (39.1809, -53.0968) (39.1438, -52.9979) (39.1061, -52.8994) (39.0678, -52.8011) (39.029, -52.7032) (38.9896, -52.6056) (38.9497, -52.5084) (38.9091, -52.4115) (38.8708, -52.3218) (38.8403, -52.2516) (38.818, -52.2009) (38.8039, -52.1693) (38.7984, -52.1569) knots -1 -1 -1 -1 -1 -1 -0.985714 -0.971429 -0.957143 -0.942857 -0.928571 -0.914286 -0.9 -0.885714 -0.871429 -0.857143 -0.842857 -0.828571 -0.814286 -0.8 -0.785714 -0.771429 -0.757143 -0.742857 -0.728571 -0.714286 -0.7 -0.685714 -0.671429 -0.657143 -0.642857 -0.628571 -0.614286 -0.6 -0.585714 -0.571429 -0.557143 -0.542857 -0.528571 -0.514286 -0.5 -0.485714 -0.471429 -0.457143 -0.442857 -0.428571 -0.414286 -0.4 -0.385714 -0.371429 -0.357143 -0.342857 -0.328571 -0.314286 -0.3 -0.285714 -0.271429 -0.257143 -0.242857 -0.228571 -0.21931 -0.21931 -0.21931 -0.21931 -0.21931 -0.21931
  spline S155 degree 3 poles (39.2465, -50.363) (39.0924, -50.4831) (38.9633, -50.6321) (38.7693, -50.9712) (38.7064, -51.1581) (38.6633, -51.4882) (38.6643, -51.6263) (38.704, -51.8986) (38.7424, -52.0313) (38.7984, -52.1569) knots 0 0 0 0 0.058597 0.058597 0.117193 0.117193 0.158456 0.158456 0.199718 0.199718 0.199718 0.199718
  arc A78 (39.2465, -50.363) -> (39.3725, -50.2646) centre (0, 0) ccw
  spline S156 degree 3 poles (41.2214, -50.2638) (41.0676, -50.1435) (40.8917, -50.0544) (40.5156, -49.9486) (40.3191, -49.9329) (39.9884, -49.9712) (39.8546, -50.0057) (39.6002, -50.1103) (39.4807, -50.1798) (39.3725, -50.2646) knots 0 0 0 0 0.058597 0.058597 0.117193 0.117193 0.158456 0.158456 0.199718 0.199718 0.199718 0.199718
  spline S157 degree 5 poles (41.2214, -50.2638) (41.2321, -50.2722) (41.2594, -50.2934) (41.3032, -50.3274) (41.3639, -50.374) (41.4417, -50.4328) (41.5259, -50.4956) (41.6106, -50.5579) (41.6957, -50.6197) (41.7813, -50.6811) (41.8674, -50.742) (41.9539, -50.8024) (42.0409, -50.8623) (42.1283, -50.9218) (42.2161, -50.9809) (42.3043, -51.0395) (42.3929, -51.0977) (42.482, -51.1555) (42.5714, -51.2128) (42.6612, -51.2697) (42.7513, -51.3263) (42.8419, -51.3824) (42.9328, -51.4381) (43.0241, -51.4934) (43.1157, -51.5483) (43.2076, -51.6028) (43.2999, -51.657) (43.3926, -51.7107) (43.4856, -51.7641) (43.5789, -51.8171) (43.6725, -51.8697) (43.7665, -51.9219) (43.8607, -51.9738) (43.9553, -52.0253) (44.0502, -52.0764) (44.1454, -52.1272) (44.2409, -52.1776) (44.3367, -52.2277) (44.4328, -52.2774) (44.5292, -52.3267) (44.6258, -52.3757) (44.7228, -52.4243) (44.82, -52.4726) (44.9175, -52.5206) (45.0153, -52.5682) (45.1134, -52.6155) (45.2117, -52.6624) (45.3103, -52.709) (45.4092, -52.7552) (45.5083, -52.8011) (45.6077, -52.8467) (45.7073, -52.8919) (45.8072, -52.9368) (45.9073, -52.9814) (46.0077, -53.0256) (46.1084, -53.0695) (46.1891, -53.1044) (46.2497, -53.1304) (46.2902, -53.1477) (46.3105, -53.1563) knots 0.21931 0.21931 0.21931 0.21931 0.21931 0.21931 0.228571 0.242857 0.257143 0.271429 0.285714 0.3 0.314286 0.328571 0.342857 0.357143 0.371429 0.385714 0.4 0.414286 0.428571 0.442857 0.457143 0.471429 0.485714 0.5 0.514286 0.528571 0.542857 0.557143 0.571429 0.585714 0.6 0.614286 0.628571 0.642857 0.657143 0.671429 0.685714 0.7 0.714286 0.728571 0.742857 0.757143 0.771429 0.785714 0.8 0.814286 0.828571 0.842857 0.857143 0.871429 0.885714 0.9 0.914286 0.928571 0.942857 0.957143 0.971429 0.985714 1 1 1 1 1 1
  arc A79 (46.3105, -53.1563) -> (48.0243, -51.6131) centre (0, 0) ccw
  spline S158 degree 5 poles (48.0243, -51.6131) (48.0179, -51.5921) (48.0049, -51.55) (47.9854, -51.487) (47.9592, -51.4031) (47.926, -51.2984) (47.8925, -51.1939) (47.8587, -51.0897) (47.8244, -50.9856) (47.7899, -50.8818) (47.7549, -50.7782) (47.7196, -50.6748) (47.684, -50.5717) (47.648, -50.4688) (47.6116, -50.3661) (47.5748, -50.2636) (47.5377, -50.1614) (47.5002, -50.0594) (47.4624, -49.9576) (47.4241, -49.8561) (47.3855, -49.7549) (47.3465, -49.6539) (47.3071, -49.5531) (47.2673, -49.4526) (47.2272, -49.3524) (47.1866, -49.2524) (47.1457, -49.1527) (47.1044, -49.0532) (47.0626, -48.954) (47.0205, -48.8551) (46.978, -48.7565) (46.935, -48.6582) (46.8917, -48.5601) (46.8479, -48.4624) (46.8037, -48.3649) (46.7591, -48.2677) (46.7141, -48.1709) (46.6686, -48.0743) (46.6227, -47.9781) (46.5764, -47.8822) (46.5296, -47.7866) (46.4823, -47.6914) (46.4347, -47.5964) (46.3865, -47.5019) (46.3379, -47.4076) (46.2888, -47.3138) (46.2393, -47.2203) (46.1892, -47.1271) (46.1387, -47.0344) (46.0877, -46.942) (46.0361, -46.8501) (45.9841, -46.7585) (45.9315, -46.6674) (45.8784, -46.5766) (45.8247, -46.4863) (45.7743, -46.4028) (45.7344, -46.3376) (45.7051, -46.2904) (45.6869, -46.2611) (45.6797, -46.2496) knots -1 -1 -1 -1 -1 -1 -0.985714 -0.971429 -0.957143 -0.942857 -0.928571 -0.914286 -0.9 -0.885714 -0.871429 -0.857143 -0.842857 -0.828571 -0.814286 -0.8 -0.785714 -0.771429 -0.757143 -0.742857 -0.728571 -0.714286 -0.7 -0.685714 -0.671429 -0.657143 -0.642857 -0.628571 -0.614286 -0.6 -0.585714 -0.571429 -0.557143 -0.542857 -0.528571 -0.514286 -0.5 -0.485714 -0.471429 -0.457143 -0.442857 -0.428571 -0.414286 -0.4 -0.385714 -0.371429 -0.357143 -0.342857 -0.328571 -0.314286 -0.3 -0.285714 -0.271429 -0.257143 -0.242857 -0.228571 -0.21931 -0.21931 -0.21931 -0.21931 -0.21931 -0.21931
  spline S159 degree 3 poles (45.8737, -44.4109) (45.7378, -44.5512) (45.6307, -44.7167) (45.4859, -45.0795) (45.4496, -45.2733) (45.4528, -45.6062) (45.473, -45.7429) (45.5502, -46.0069) (45.6067, -46.133) (45.6797, -46.2496) knots 0 0 0 0 0.058597 0.058597 0.117193 0.117193 0.158456 0.158456 0.199718 0.199718 0.199718 0.199718
  arc A80 (45.8737, -44.4109) -> (45.9848, -44.2958) centre (0, 0) ccw
  spline S160 degree 3 poles (47.8157, -44.0378) (47.6465, -43.94) (47.46, -43.8763) (47.0729, -43.8238) (46.876, -43.8357) (46.5539, -43.9196) (46.4262, -43.9724) (46.1888, -44.1113) (46.0802, -44.1968) (45.9848, -44.2958) knots 0 0 0 0 0.058597 0.058597 0.117193 0.117193 0.158456 0.158456 0.199718 0.199718 0.199718 0.199718
  spline S161 degree 5 poles (47.8157, -44.0378) (47.8274, -44.0446) (47.8573, -44.0618) (47.9055, -44.0893) (47.9721, -44.127) (48.0573, -44.1745) (48.1494, -44.2249) (48.2419, -44.2748) (48.3348, -44.3242) (48.4282, -44.373) (48.5219, -44.4213) (48.6159, -44.4691) (48.7104, -44.5164) (48.8052, -44.5632) (48.9004, -44.6094) (48.9959, -44.6552) (49.0918, -44.7005) (49.188, -44.7453) (49.2845, -44.7896) (49.3814, -44.8335) (49.4785, -44.8769) (49.576, -44.9199) (49.6738, -44.9624) (49.7718, -45.0045) (49.8702, -45.0461) (49.9689, -45.0873) (50.0678, -45.128) (50.167, -45.1684) (50.2665, -45.2083) (50.3663, -45.2478) (50.4664, -45.2868) (50.5667, -45.3255) (50.6673, -45.3637) (50.7681, -45.4016) (50.8692, -45.439) (50.9705, -45.476) (51.0721, -45.5127) (51.1739, -45.5489) (51.276, -45.5848) (51.3783, -45.6202) (51.4808, -45.6553) (51.5836, -45.6899) (51.6866, -45.7242) (51.7899, -45.7582) (51.8933, -45.7917) (51.997, -45.8248) (52.1009, -45.8576) (52.205, -45.89) (52.3094, -45.9221) (52.4139, -45.9537) (52.5187, -45.985) (52.6236, -46.0159) (52.7288, -46.0465) (52.8342, -46.0767) (52.9397, -46.1065) (53.0455, -46.136) (53.1303, -46.1593) (53.194, -46.1766) (53.2364, -46.1881) (53.2577, -46.1938) knots 0.21931 0.21931 0.21931 0.21931 0.21931 0.21931 0.228571 0.242857 0.257143 0.271429 0.285714 0.3 0.314286 0.328571 0.342857 0.357143 0.371429 0.385714 0.4 0.414286 0.428571 0.442857 0.457143 0.471429 0.485714 0.5 0.514286 0.528571 0.542857 0.557143 0.571429 0.585714 0.6 0.614286 0.628571 0.642857 0.657143 0.671429 0.685714 0.7 0.714286 0.728571 0.742857 0.757143 0.771429 0.785714 0.8 0.814286 0.828571 0.842857 0.857143 0.871429 0.885714 0.9 0.914286 0.928571 0.942857 0.957143 0.971429 0.985714 1 1 1 1 1 1
  arc A81 (53.2577, -46.1938) -> (54.7401, -44.4271) centre (0, 0) ccw
  spline S162 degree 5 poles (54.7401, -44.4271) (54.7308, -44.4072) (54.7121, -44.3673) (54.684, -44.3076) (54.6464, -44.2282) (54.599, -44.1291) (54.5512, -44.0304) (54.5032, -43.9318) (54.4548, -43.8336) (54.4062, -43.7356) (54.3572, -43.6378) (54.3078, -43.5404) (54.2582, -43.4432) (54.2082, -43.3463) (54.1578, -43.2496) (54.1072, -43.1533) (54.0562, -43.0572) (54.0049, -42.9615) (53.9532, -42.866) (53.9012, -42.7708) (53.8489, -42.6759) (53.7962, -42.5813) (53.7432, -42.487) (53.6898, -42.393) (53.6361, -42.2993) (53.582, -42.2059) (53.5276, -42.1129) (53.4728, -42.0202) (53.4177, -41.9278) (53.3622, -41.8357) (53.3064, -41.744) (53.2502, -41.6525) (53.1936, -41.5615) (53.1366, -41.4708) (53.0793, -41.3804) (53.0216, -41.2904) (52.9635, -41.2007) (52.9051, -41.1115) (52.8462, -41.0226) (52.787, -40.934) (52.7274, -40.8459) (52.6673, -40.7581) (52.6069, -40.6708) (52.5461, -40.5838) (52.4848, -40.4973) (52.4232, -40.4111) (52.3611, -40.3254) (52.2986, -40.2402) (52.2356, -40.1554) (52.1722, -40.071) (52.1084, -39.9871) (52.0441, -39.9037) (51.9793, -39.8208) (51.9141, -39.7383) (51.8484, -39.6564) (51.7869, -39.5807) (51.7382, -39.5217) (51.7027, -39.479) (51.6806, -39.4525) (51.6718, -39.4422) knots -1 -1 -1 -1 -1 -1 -0.985714 -0.971429 -0.957143 -0.942857 -0.928571 -0.914286 -0.9 -0.885714 -0.871429 -0.857143 -0.842857 -0.828571 -0.814286 -0.8 -0.785714 -0.771429 -0.757143 -0.742857 -0.728571 -0.714286 -0.7 -0.685714 -0.671429 -0.657143 -0.642857 -0.628571 -0.614286 -0.6 -0.585714 -0.571429 -0.557143 -0.542857 -0.528571 -0.514286 -0.5 -0.485714 -0.471429 -0.457143 -0.442857 -0.428571 -0.414286 -0.4 -0.385714 -0.371429 -0.357143 -0.342857 -0.328571 -0.314286 -0.3 -0.285714 -0.271429 -0.257143 -0.242857 -0.228571 -0.21931 -0.21931 -0.21931 -0.21931 -0.21931 -0.21931
  spline S163 degree 3 poles (51.6081, -37.5943) (51.493, -37.7521) (51.41, -37.931) (51.3171, -38.3104) (51.3081, -38.5074) (51.3576, -38.8365) (51.3967, -38.9691) (51.5098, -39.2198) (51.5834, -39.3368) (51.6718, -39.4422) knots 0 0 0 0 0.058597 0.058597 0.117193 0.117193 0.158456 0.158456 0.199718 0.199718 0.199718 0.199718
  arc A82 (51.6081, -37.5943) -> (51.702, -37.4649) centre (0, 0) ccw
  spline S164 degree 3 poles (53.4792, -36.9545) (53.2981, -36.8813) (53.1045, -36.8441) (52.7138, -36.8461) (52.5206, -36.8852) (52.2133, -37.0131) (52.0942, -37.0832) (51.8784, -37.2538) (51.7827, -37.3535) (51.702, -37.4649) knots 0 0 0 0 0.058597 0.058597 0.117193 0.117193 0.158456 0.158456 0.199718 0.199718 0.199718 0.199718
  spline S165 degree 5 poles (53.4792, -36.9545) (53.4918, -36.9596) (53.5238, -36.9725) (53.5753, -36.9931) (53.6465, -37.0211) (53.7375, -37.0563) (53.8357, -37.0934) (53.9343, -37.13) (54.0332, -37.1659) (54.1324, -37.2013) (54.2319, -37.2361) (54.3317, -37.2703) (54.4318, -37.304) (54.5322, -37.3371) (54.6329, -37.3697) (54.7339, -37.4017) (54.8351, -37.4332) (54.9366, -37.4642) (55.0384, -37.4947) (55.1404, -37.5246) (55.2427, -37.5541) (55.3452, -37.5831) (55.4479, -37.6116) (55.5509, -37.6396) (55.6541, -37.6671) (55.7575, -37.6942) (55.8612, -37.7208) (55.965, -37.7469) (56.0691, -37.7726) (56.1734, -37.7978) (56.2779, -37.8225) (56.3827, -37.8469) (56.4876, -37.8707) (56.5927, -37.8942) (56.698, -37.9172) (56.8035, -37.9398) (56.9092, -37.9619) (57.0151, -37.9836) (57.1211, -38.0049) (57.2274, -38.0258) (57.3338, -38.0462) (57.4404, -38.0662) (57.5472, -38.0859) (57.6541, -38.1051) (57.7613, -38.1239) (57.8686, -38.1423) (57.976, -38.1603) (58.0836, -38.1779) (58.1914, -38.1951) (58.2993, -38.2119) (58.4074, -38.2283) (58.5157, -38.2443) (58.6241, -38.2599) (58.7326, -38.2752) (58.8413, -38.29) (58.9502, -38.3045) (59.0374, -38.3158) (59.1028, -38.3241) (59.1465, -38.3295) (59.1683, -38.3322) knots 0.21931 0.21931 0.21931 0.21931 0.21931 0.21931 0.228571 0.242857 0.257143 0.271429 0.285714 0.3 0.314286 0.328571 0.342857 0.357143 0.371429 0.385714 0.4 0.414286 0.428571 0.442857 0.457143 0.471429 0.485714 0.5 0.514286 0.528571 0.542857 0.557143 0.571429 0.585714 0.6 0.614286 0.628571 0.642857 0.657143 0.671429 0.685714 0.7 0.714286 0.728571 0.742857 0.757143 0.771429 0.785714 0.8 0.814286 0.828571 0.842857 0.857143 0.871429 0.885714 0.9 0.914286 0.928571 0.942857 0.957143 0.971429 0.985714 1 1 1 1 1 1
  arc A83 (59.1683, -38.3322) -> (60.3905, -36.3764) centre (0, 0) ccw
  spline S166 degree 5 poles (60.3905, -36.3764) (60.3785, -36.358) (60.3544, -36.3211) (60.3183, -36.2659) (60.2699, -36.1925) (60.2092, -36.101) (60.1482, -36.0098) (60.0869, -35.9189) (60.0253, -35.8283) (59.9635, -35.7381) (59.9014, -35.6481) (59.8389, -35.5585) (59.7762, -35.4691) (59.7132, -35.3801) (59.65, -35.2914) (59.5864, -35.2031) (59.5225, -35.115) (59.4584, -35.0273) (59.3939, -34.94) (59.3292, -34.8529) (59.2642, -34.7662) (59.1988, -34.6799) (59.1332, -34.5939) (59.0673, -34.5082) (59.001, -34.423) (58.9345, -34.338) (58.8677, -34.2535) (58.8005, -34.1693) (58.7331, -34.0854) (58.6653, -34.002) (58.5972, -33.9189) (58.5288, -33.8362) (58.4601, -33.7539) (58.3911, -33.672) (58.3218, -33.5905) (58.2521, -33.5094) (58.1821, -33.4287) (58.1118, -33.3484) (58.0412, -33.2686) (57.9702, -33.1891) (57.8989, -33.1102) (57.8272, -33.0316) (57.7552, -32.9535) (57.6829, -32.8759) (57.6102, -32.7987) (57.5371, -32.722) (57.4637, -32.6457) (57.3899, -32.57) (57.3158, -32.4948) (57.2413, -32.4201) (57.1664, -32.3459) (57.0911, -32.2722) (57.0154, -32.1991) (56.9394, -32.1265) (56.8629, -32.0545) (56.7915, -31.9881) (56.7351, -31.9365) (56.694, -31.8992) (56.6683, -31.8761) (56.6583, -31.867) knots -1 -1 -1 -1 -1 -1 -0.985714 -0.971429 -0.957143 -0.942857 -0.928571 -0.914286 -0.9 -0.885714 -0.871429 -0.857143 -0.842857 -0.828571 -0.814286 -0.8 -0.785714 -0.771429 -0.757143 -0.742857 -0.728571 -0.714286 -0.7 -0.685714 -0.671429 -0.657143 -0.642857 -0.628571 -0.614286 -0.6 -0.585714 -0.571429 -0.557143 -0.542857 -0.528571 -0.514286 -0.5 -0.485714 -0.471429 -0.457143 -0.442857 -0.428571 -0.414286 -0.4 -0.385714 -0.371429 -0.357143 -0.342857 -0.328571 -0.314286 -0.3 -0.285714 -0.271429 -0.257143 -0.242857 -0.228571 -0.21931 -0.21931 -0.21931 -0.21931 -0.21931 -0.21931
  spline S167 degree 3 poles (56.3379, -30.046) (56.246, -30.2183) (56.1886, -30.4069) (56.1494, -30.7956) (56.168, -30.9919) (56.2628, -31.311) (56.3199, -31.4368) (56.4669, -31.6694) (56.556, -31.775) (56.6583, -31.867) knots 0 0 0 0 0.058597 0.058597 0.117193 0.117193 0.158456 0.158456 0.199718 0.199718 0.199718 0.199718
  arc A84 (56.3379, -30.046) -> (56.413, -29.9048) centre (0, 0) ccw
  spline S168 degree 3 poles (58.1018, -29.152) (57.9123, -29.1047) (57.7154, -29.0948) (57.3288, -29.1511) (57.1429, -29.2168) (56.8564, -29.3862) (56.7482, -29.4722) (56.5582, -29.6712) (56.4774, -29.7832) (56.413, -29.9048) knots 0 0 0 0 0.058597 0.058597 0.117193 0.117193 0.158456 0.158456 0.199718 0.199718 0.199718 0.199718
  spline S169 degree 5 poles (58.1018, -29.152) (58.115, -29.1553) (58.1485, -29.1636) (58.2024, -29.1769) (58.2767, -29.1947) (58.3717, -29.2168) (58.4742, -29.24) (58.5769, -29.2624) (58.6798, -29.2843) (58.783, -29.3055) (58.8864, -29.3261) (58.99, -29.3461) (59.0938, -29.3655) (59.1979, -29.3843) (59.3021, -29.4026) (59.4065, -29.4202) (59.5112, -29.4373) (59.616, -29.4539) (59.721, -29.4699) (59.8262, -29.4854) (59.9316, -29.5003) (60.0371, -29.5148) (60.1428, -29.5287) (60.2487, -29.5421) (60.3547, -29.555) (60.4609, -29.5674) (60.5672, -29.5793) (60.6737, -29.5907) (60.7804, -29.6017) (60.8872, -29.6121) (60.9941, -29.6221) (61.1012, -29.6316) (61.2084, -29.6406) (61.3158, -29.6492) (61.4233, -29.6573) (61.5309, -29.665) (61.6386, -29.6722) (61.7465, -29.679) (61.8545, -29.6853) (61.9626, -29.6912) (62.0709, -29.6966) (62.1792, -29.7016) (62.2877, -29.7062) (62.3963, -29.7103) (62.505, -29.7141) (62.6138, -29.7173) (62.7227, -29.7202) (62.8317, -29.7227) (62.9408, -29.7247) (63.05, -29.7263) (63.1594, -29.7275) (63.2688, -29.7283) (63.3783, -29.7287) (63.4879, -29.7287) (63.5976, -29.7283) (63.7074, -29.7275) (63.7953, -29.7265) (63.8613, -29.7256) (63.9053, -29.7249) (63.9273, -29.7245) knots 0.21931 0.21931 0.21931 0.21931 0.21931 0.21931 0.228571 0.242857 0.257143 0.271429 0.285714 0.3 0.314286 0.328571 0.342857 0.357143 0.371429 0.385714 0.4 0.414286 0.428571 0.442857 0.457143 0.471429 0.485714 0.5 0.514286 0.528571 0.542857 0.557143 0.571429 0.585714 0.6 0.614286 0.628571 0.642857 0.657143 0.671429 0.685714 0.7 0.714286 0.728571 0.742857 0.757143 0.771429 0.785714 0.8 0.814286 0.828571 0.842857 0.857143 0.871429 0.885714 0.9 0.914286 0.928571 0.942857 0.957143 0.971429 0.985714 1 1 1 1 1 1
  arc A85 (63.9273, -29.7245) -> (64.8654, -27.6177) centre (0, 0) ccw
  spline S170 degree 5 poles (64.8654, -27.6177) (64.8509, -27.6011) (64.822, -27.5679) (64.7785, -27.5183) (64.7204, -27.4523) (64.6475, -27.3701) (64.5744, -27.2883) (64.5011, -27.2069) (64.4275, -27.1257) (64.3537, -27.045) (64.2797, -26.9645) (64.2054, -26.8844) (64.1309, -26.8047) (64.0561, -26.7253) (63.9811, -26.6463) (63.9058, -26.5677) (63.8303, -26.4894) (63.7546, -26.4114) (63.6786, -26.3339) (63.6024, -26.2567) (63.5259, -26.1799) (63.4492, -26.1035) (63.3723, -26.0275) (63.2951, -25.9518) (63.2176, -25.8766) (63.1399, -25.8018) (63.0619, -25.7273) (62.9837, -25.6533) (62.9053, -25.5796) (62.8265, -25.5064) (62.7476, -25.4336) (62.6683, -25.3613) (62.5889, -25.2893) (62.5091, -25.2178) (62.4291, -25.1468) (62.3488, -25.0761) (62.2683, -25.006) (62.1875, -24.9363) (62.1064, -24.867) (62.0251, -24.7983) (61.9434, -24.73) (61.8616, -24.6621) (61.7794, -24.5948) (61.6969, -24.528) (61.6142, -24.4617) (61.5312, -24.3959) (61.4479, -24.3306) (61.3643, -24.2659) (61.2804, -24.2017) (61.1962, -24.1381) (61.1117, -24.0751) (61.0269, -24.0126) (60.9418, -23.9507) (60.8564, -23.8894) (60.7707, -23.8288) (60.6907, -23.773) (60.6276, -23.7297) (60.5817, -23.6985) (60.5531, -23.6791) (60.5419, -23.6715) knots -1 -1 -1 -1 -1 -1 -0.985714 -0.971429 -0.957143 -0.942857 -0.928571 -0.914286 -0.9 -0.885714 -0.871429 -0.857143 -0.842857 -0.828571 -0.814286 -0.8 -0.785714 -0.771429 -0.757143 -0.742857 -0.728571 -0.714286 -0.7 -0.685714 -0.671429 -0.657143 -0.642857 -0.628571 -0.614286 -0.6 -0.585714 -0.571429 -0.557143 -0.542857 -0.528571 -0.514286 -0.5 -0.485714 -0.471429 -0.457143 -0.442857 -0.428571 -0.414286 -0.4 -0.385714 -0.371429 -0.357143 -0.342857 -0.328571 -0.314286 -0.3 -0.285714 -0.271429 -0.257143 -0.242857 -0.228571 -0.21931 -0.21931 -0.21931 -0.21931 -0.21931 -0.21931
  spline S171 degree 3 poles (59.9712, -21.9128) (59.9042, -22.0963) (59.8736, -22.2911) (59.8889, -22.6814) (59.9346, -22.8732) (60.0729, -23.176) (60.147, -23.2927) (60.3249, -23.5025) (60.4278, -23.5947) (60.5419, -23.6715) knots 0 0 0 0 0.058597 0.058597 0.117193 0.117193 0.158456 0.158456 0.199718 0.199718 0.199718 0.199718
  arc A86 (59.9712, -21.9128) -> (60.0259, -21.7626) centre (0, 0) ccw
  spline S172 degree 3 poles (61.5935, -20.7821) (61.3993, -20.7616) (61.2029, -20.7793) (60.8279, -20.8888) (60.653, -20.9797) (60.3928, -21.1873) (60.2976, -21.2875) (60.1372, -21.511) (60.0728, -21.6333) (60.0259, -21.7626) knots 0 0 0 0 0.058597 0.058597 0.117193 0.117193 0.158456 0.158456 0.199718 0.199718 0.199718 0.199718
  spline S173 degree 5 poles (61.5935, -20.7821) (61.607, -20.7835) (61.6414, -20.7871) (61.6966, -20.7927) (61.7727, -20.8) (61.8699, -20.8087) (61.9745, -20.8174) (62.0794, -20.8253) (62.1844, -20.8326) (62.2895, -20.8393) (62.3947, -20.8453) (62.5001, -20.8507) (62.6056, -20.8554) (62.7113, -20.8596) (62.817, -20.8632) (62.9229, -20.8661) (63.0289, -20.8685) (63.135, -20.8703) (63.2412, -20.8715) (63.3475, -20.8722) (63.454, -20.8724) (63.5605, -20.872) (63.6671, -20.8711) (63.7738, -20.8696) (63.8806, -20.8676) (63.9875, -20.8651) (64.0945, -20.8621) (64.2015, -20.8586) (64.3086, -20.8546) (64.4159, -20.8501) (64.5231, -20.8451) (64.6305, -20.8396) (64.7379, -20.8336) (64.8454, -20.8272) (64.953, -20.8202) (65.0606, -20.8129) (65.1683, -20.805) (65.2761, -20.7967) (65.3839, -20.7879) (65.4918, -20.7787) (65.5998, -20.769) (65.7078, -20.7589) (65.8158, -20.7483) (65.9239, -20.7373) (66.0321, -20.7259) (66.1403, -20.714) (66.2485, -20.7017) (66.3568, -20.6889) (66.4652, -20.6758) (66.5735, -20.6622) (66.682, -20.6481) (66.7904, -20.6337) (66.8989, -20.6188) (67.0075, -20.6036) (67.1161, -20.5879) (67.2247, -20.5718) (67.3116, -20.5586) (67.3768, -20.5485) (67.4203, -20.5417) (67.442, -20.5383) knots 0.21931 0.21931 0.21931 0.21931 0.21931 0.21931 0.228571 0.242857 0.257143 0.271429 0.285714 0.3 0.314286 0.328571 0.342857 0.357143 0.371429 0.385714 0.4 0.414286 0.428571 0.442857 0.457143 0.471429 0.485714 0.5 0.514286 0.528571 0.542857 0.557143 0.571429 0.585714 0.6 0.614286 0.628571 0.642857 0.657143 0.671429 0.685714 0.7 0.714286 0.728571 0.742857 0.757143 0.771429 0.785714 0.8 0.814286 0.828571 0.842857 0.857143 0.871429 0.885714 0.9 0.914286 0.928571 0.942857 0.957143 0.971429 0.985714 1 1 1 1 1 1
  arc A87 (67.442, -20.5383) -> (68.0777, -18.3214) centre (0, 0) ccw
  spline S174 degree 5 poles (68.0777, -18.3214) (68.0611, -18.307) (68.0278, -18.2781) (67.9779, -18.235) (67.9112, -18.1778) (67.8276, -18.1066) (67.7438, -18.0357) (67.6598, -17.9653) (67.5757, -17.8952) (67.4914, -17.8254) (67.4068, -17.7561) (67.3221, -17.6871) (67.2372, -17.6185) (67.1521, -17.5503) (67.0669, -17.4825) (66.9814, -17.4151) (66.8957, -17.3481) (66.8099, -17.2815) (66.7239, -17.2153) (66.6377, -17.1494) (66.5512, -17.084) (66.4646, -17.019) (66.3779, -16.9545) (66.2909, -16.8903) (66.2037, -16.8266) (66.1163, -16.7633) (66.0288, -16.7004) (65.941, -16.638) (65.8531, -16.576) (65.7649, -16.5144) (65.6766, -16.4533) (65.5881, -16.3927) (65.4993, -16.3325) (65.4104, -16.2728) (65.3213, -16.2136) (65.232, -16.1548) (65.1425, -16.0965) (65.0527, -16.0388) (64.9628, -15.9815) (64.8727, -15.9247) (64.7824, -15.8684) (64.6918, -15.8127) (64.6011, -15.7574) (64.5102, -15.7027) (64.419, -15.6486) (64.3276, -15.595) (64.2361, -15.542) (64.1443, -15.4895) (64.0523, -15.4376) (63.96, -15.3864) (63.8676, -15.3357) (63.7749, -15.2856) (63.682, -15.2362) (63.5889, -15.1874) (63.4956, -15.1392) (63.4086, -15.0951) (63.3401, -15.061) (63.2904, -15.0365) (63.2593, -15.0213) (63.2471, -15.0154) knots -1 -1 -1 -1 -1 -1 -0.985714 -0.971429 -0.957143 -0.942857 -0.928571 -0.914286 -0.9 -0.885714 -0.871429 -0.857143 -0.842857 -0.828571 -0.814286 -0.8 -0.785714 -0.771429 -0.757143 -0.742857 -0.728571 -0.714286 -0.7 -0.685714 -0.671429 -0.657143 -0.642857 -0.628571 -0.614286 -0.6 -0.585714 -0.571429 -0.557143 -0.542857 -0.528571 -0.514286 -0.5 -0.485714 -0.471429 -0.457143 -0.442857 -0.428571 -0.414286 -0.4 -0.385714 -0.371429 -0.357143 -0.342857 -0.328571 -0.314286 -0.3 -0.285714 -0.271429 -0.257143 -0.242857 -0.228571 -0.21931 -0.21931 -0.21931 -0.21931 -0.21931 -0.21931
  spline S175 degree 3 poles (62.4373, -13.3532) (62.3964, -13.5442) (62.3933, -13.7413) (62.4627, -14.1258) (62.5347, -14.3094) (62.7138, -14.5899) (62.8034, -14.6951) (63.0087, -14.8782) (63.1235, -14.9551) (63.2471, -15.0154) knots 0 0 0 0 0.058597 0.058597 0.117193 0.117193 0.158456 0.158456 0.199718 0.199718 0.199718 0.199718
  arc A88 (62.4373, -13.3532) -> (62.4705, -13.1968) centre (0, 0) ccw